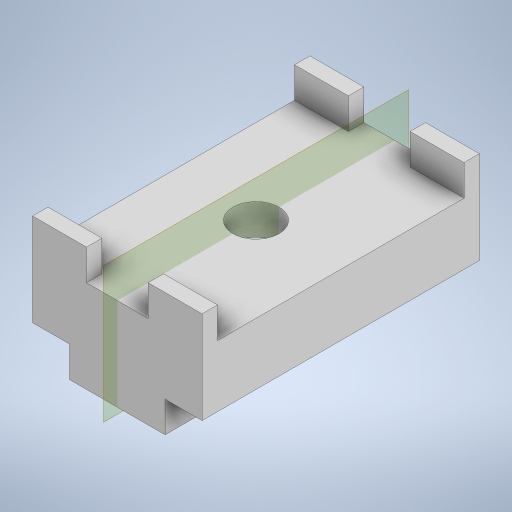
# Autodesk Inventor part: Bartosz_Zukowski_model_nr_5_1
Saved by Autodesk Inventor 2024 (Build 280153000, 153)
## iProperties
Created: 2024-03-20
Part Number: Bartosz_Zukowski_model_nr_5_1
Material: Ogólny
Document SubType Name: Modeling
Designer: student156p
Density: 1 g/cm^3
Appearance: Domyślna
Author: student156p
Autodesk Inventor part; units mm, degrees
ref_plane "YZ Plane" through (0, 0, 0) normal (1, 0, 0) x (0, 1, 0)
ref_plane "XZ Plane" through (0, 0, 0) normal (0, 1, 0) x (-1, 0, 0)
ref_plane "XY Plane" through (0, 0, 0) normal (0, 0, 1) x (1, 0, 0)
sketch "Szkic1" plane through (0, 0, 0) normal (0, 0, 1) x (1, 0, 0)
  line L0 (-27.5, 10.1009) -> (-10, 10.1009)
  line L1 (-10, 10.1009) -> (-10, 0.1009)
  line L2 (-10, 0.1009) -> (10, 0.1009)
  line L3 (-27.5, 10.1009) -> (-27.5, -19.8991)
  line L4 (-27.5, -19.8991) -> (-15.5, -19.8991)
  line L5 (-15.5, -19.8991) -> (-15.5, -29.8991)
  line L6 (-15.5, -29.8991) -> (15.5, -29.8991)
  line L7 (27.5, 10.1009) -> (10, 10.1009)
  line L8 (10, 10.1009) -> (10, 0.1009)
  line L9 (27.5, 10.1009) -> (27.5, -19.8991)
  line L10 (27.5, -19.8991) -> (15.5, -19.8991)
  line L11 (15.5, -19.8991) -> (15.5, -29.8991)
  point P0 (0, 0)
  dimension "d1" = 55
  dimension "d2" = 17.5
  dimension "d3" = 20
  dimension "d4" = 12
  dimension "d5" = 12
  dimension "d6" = 10
  dimension "d14" = 40
  dimension "d15" = 40
  dimension "d16" = 10
  dimension "d17" = 10
  constraints: 24 end point, 4 perpendicular, 2 horizontal, 1 vertical
  measures "d1" distance between parallel lines of L9 L3
  measures "d2" distance of L0.start L0.end
  measures "d3" distance between parallel lines of L8 L1
  measures "d4" distance of L3.end L4.end
  measures "d5" distance of L9.end L10.end
  measures "d6" distance of L4.end L5.end
  measures "d14" distance between parallel lines of L6 L7
  measures "d15" distance between parallel lines of L6 L0
  measures "d16" distance between parallel lines of L2 L7
  measures "d17" distance between parallel lines of L6 L10
extrude "Wyciągnięcie proste1" add sketch "Szkic1" along normal blind 90
sketch "Szkic3" plane through (-27.5, -19.8991, 0) normal (-1, 0, 0) x (0, 0, 1)
  line L0 (5, 30) -> (85, 30)
  line L1 (85, 30) -> (85, 20)
  line L2 (85, 20) -> (5, 20)
  line L3 (5, 20) -> (5, 30)
  line L4 (0, 30) -> (0, 0) projected
  line L5 (0, 30) -> (90, 30) projected
  point P0 (0, 19.8991)
  dimension "d19" = 5
  dimension "d20" = 10
  constraints: 8 end point, 2 parallel, 1 collinear, 1 horizontal, 1 perpendicular
  measures "d19" distance between parallel lines of L3 L4
  measures "d20" distance of L2.end L0.start
extrude "Wyciągnięcie proste3" cut sketch "Szkic3" against normal through all
sketch "Szkic4" plane through (-15.5, -29.8991, 0) normal (-1, 0, 0) x (0, 0, 1)
  line L0 (20, 0) -> (70, 0)
  line L1 (70, 0) -> (70, 10)
  line L2 (70, 10) -> (20, 10)
  line L3 (20, 10) -> (20, 0)
  line L4 (0, 10) -> (0, 0) projected
  point P0 (0, 29.8991)
  dimension "d23" = 20
  dimension "d24" = 50
  constraints: 8 end point, 2 parallel, 1 horizontal, 1 perpendicular
  measures "d23" distance between parallel lines of L4 L3
  measures "d24" distance of L0.start L0.end
extrude "Wyciągnięcie proste4" cut sketch "Szkic4" against normal through all
sketch "Szkic5" plane through (-10, 0.1009, 0) normal (0, 1, 0) x (1, 0, 0)
  line L0 (0, -85) -> (0, -90) construction
  line L1 (20, -90) -> (0, -90) construction
  line L2 (20, -85) -> (20, -90) construction
  line L3 (20, -85) -> (37.5, -85) construction
  line L4 (37.5, -5) -> (37.5, -85) construction
  line L5 (20, -5) -> (37.5, -5) construction
  line L6 (20, 0) -> (20, -5) construction
  line L7 (20, 0) -> (0, 0) construction
  line L8 (0, 0) -> (0, -5) construction
  line L9 (-17.5, -5) -> (0, -5) construction
  line L10 (-17.5, -85) -> (-17.5, -5) construction
  line L11 (-17.5, -85) -> (0, -85) construction
  circle A0 centre (10, -45) radius 7.5
  point P0 (10, 0)
  dimension "d27" = 15
  constraints: 1 centre point
  measures "d27" diameter of A0
extrude "Wyciągnięcie proste5" cut sketch "Szkic5" against normal through all
ref_plane "Płaszczyzna konstrukcyjna1" through (0, -19.8991, 0) normal (-1, 0, 0) x (0, 0, 1)
sketch "Szkic6" plane through (0, -19.8991, 0) normal (-1, 0, 0) x (0, 0, 1)
  line L0 (85, 30) -> (85, 20) projected
  line L1 (85, 20) -> (5, 20) projected
  line L2 (5, 20) -> (5, 30) projected
  line L3 (0, 30) -> (5, 30) projected
  line L4 (0, 30) -> (0, 0) projected
  line L5 (0, 0) -> (90, 0) projected
  line L6 (90, 30) -> (90, 0) projected
  line L7 (85, 30) -> (90, 30) projected
  line L8 (70, 0) -> (20, 0)
  line L9 (20, 0) -> (20, 10)
  line L10 (20, 10) -> (70, 10)
  line L11 (70, 10) -> (70, 0)
  point P0 (0, 19.8991)
  constraints: 8 end point, 2 parallel, 1 horizontal, 1 perpendicular, 1 point on line
extrude "Wyciągnięcie proste6" cut sketch "Szkic6" along normal mid plane 35 contours L5 L9 L10 L11
